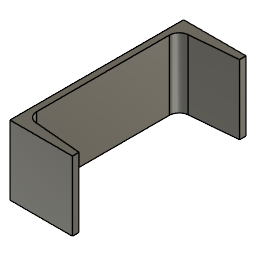
C-250×90×9×13 (Autodesk Fusion 360 design; units mm, degrees)
Autodesk Fusion 360 part; units mm, degrees
note: some values were not read from the file. Set by a fixed rule: which sketch regions a step uses.
sketch "スケッチ1" plane through (0, 0, 0) normal (0, 0, 1) x (1, 0, 0)
  arc A0 (21.7798, 234.5748) -> (9, 220.6281) centre (23, 220.6281) ccw
  line L0 (0, 250) -> (0, 0)
  line L1 (0, 0) -> (90, 0)
  line L2 (21.7798, 15.4252) -> (90, 9.4567)
  line L3 (9, 220.6281) -> (9, 29.3719)
  arc A1 (9, 29.3719) -> (21.7798, 15.4252) centre (23, 29.3719) ccw
  line L4 (90, 9.4567) -> (90, 0)
  line L5 (90, 240.5433) -> (21.7798, 234.5748)
  line L6 (0, 250) -> (90, 250)
  line L7 (90, 250) -> (90, 240.5433)
extrude "押し出し1" add sketch "スケッチ1" along normal blind 100
